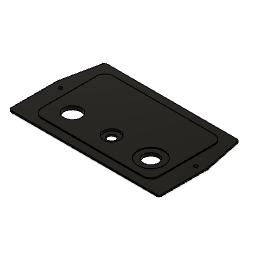
CableCover_Fusion (Autodesk Fusion 360 design; units mm, degrees)
Autodesk Fusion 360 part; units mm, degrees
sketch "Sketch1" plane through (0, 0, 0) normal (0, 1, 0) x (1, 0, 0)
  line L0 (-102.5, 67.5) -> (102.5, 67.5)
  line L1 (102.5, 67.5) -> (102.5, -67.5)
  line L2 (102.5, -67.5) -> (-102.5, -67.5)
  line L3 (-102.5, -67.5) -> (-102.5, 67.5)
  dimension "d1" = 205
  dimension "d2" = 135
  dimension "d3" = 67.5
  dimension "d4" = 102.5
  constraint horizontal L0
  constraint vertical L1
  constraint horizontal L2
  constraint vertical L3
  measures "d1" distance of L0.start L0.end
  measures "d2" distance of L0.start L2.end
  measures "d3" distance of origin L0
  measures "d4" distance of origin L1
  measures "d7" distance of L0.start
extrude "Extrude1" add sketch "Sketch1" along normal blind 10 makes body 1
sketch "Sketch2" plane through (0, 10, 0) normal (0, 1, 0) x (-1, 0, 0)
  line L0 (102.5, 67.5) -> (-102.5, 67.5)
  line L1 (-102.5, 67.5) -> (-102.5, -67.5)
  line L2 (-102.5, -67.5) -> (102.5, -67.5)
  line L3 (102.5, -67.5) -> (102.5, 67.5)
  line L4 (90, -55) -> (-90, -55)
  line L5 (-90, -55) -> (-90, 55)
  line L6 (-90, 55) -> (90, 55)
  line L7 (90, 55) -> (90, -55)
  dimension "d7" = 12.5
  dimension "d8" = 12.5
  dimension "d9" = 12.5
  dimension "d10" = 12.5
  constraint horizontal L4
  constraint vertical L5
  constraint horizontal L6
  constraint vertical L7
  measures "d7" distance of L3 L7
  measures "d8" distance of L1 L5
  measures "d9" distance of L2 L4
  measures "d10" distance of L0 L6
extrude "Extrude2" cut sketch "Sketch2" against normal blind 6 bodies 1
sketch "Sketch3" plane through (102.5, 0, 0) normal (1, 0, 0) x (0, 0, -1)
  line L0 (67.5, 4) -> (-67.5, 4)
  line L1 (-67.5, 4) -> (-67.5, 0)
  line L2 (-67.5, 0) -> (67.5, 0)
  line L3 (67.5, 0) -> (67.5, 4)
extrude "Extrude3" add sketch "Sketch3" along normal blind 12.5 bodies 1
extrude "Extrude4" add 1 faces at (-102.5, 1.3333, 22.5) along direction (-1, 0, 0) blind 12.5 on bodies 1 bodies 1
sketch "Sketch4" plane through (0, 4, 0) normal (0, 1, 0) x (-1, 0, 0)
  line L0 (-90, 55) -> (90, 55)
  line L1 (90, 55) -> (90, -55)
  line L2 (90, -55) -> (-90, -55)
  line L3 (-90, -55) -> (-90, 55)
  line L4 (115, 67.5) -> (-115, 67.5)
  line L5 (-115, 67.5) -> (-115, -67.5)
  line L6 (-115, -67.5) -> (115, -67.5)
  line L7 (115, -67.5) -> (115, 67.5)
  point P0 (103.5, 0)
  point P1 (-103.5, 0)
  dimension "d17" = 207
  dimension "d18" = 11.5
  dimension "d19" = 67.5
  dimension "d20" = 67.5
  measures "d17" horizontal distance of P0 P1
  measures "d18" distance of L7 P0
  measures "d19" distance of L4 P0
  measures "d20" distance of L4 P1
hole "Hole1" at (-103.5, 4, 0) at (103.5, 4, 0) direction (0, -1, 0) diameter 5.3 depth 4 tip angle 180 bodies 1
fillet "Fillet1" radius 12.5 4 edges at (-90, 7, -55) (-90, 7, 55) (90, 7, 55) (90, 7, -55) on bodies 1
sketch "Sketch5" plane through (0, 4, 0) normal (0, 1, 0) x (-1, 0, 0)
  circle A0 centre (103.5, 0) radius 2.65
  circle A1 centre (-103.5, 0) radius 2.65
  line L0 (90, 42.5) -> (90, -42.5)
  arc A2 (77.5, -55) -> (90, -42.5) centre (77.5, -42.5) ccw
  line L1 (77.5, -55) -> (-77.5, -55)
  arc A3 (-90, -42.5) -> (-77.5, -55) centre (-77.5, -42.5) ccw
  line L2 (-90, -42.5) -> (-90, 42.5)
  arc A4 (-77.5, 55) -> (-90, 42.5) centre (-77.5, 42.5) ccw
  line L3 (-77.5, 55) -> (77.5, 55)
  arc A5 (90, 42.5) -> (77.5, 55) centre (77.5, 42.5) ccw
  line L4 (115, 67.5) -> (-115, 67.5)
  line L5 (-115, 67.5) -> (-115, -67.5)
  line L6 (-115, -67.5) -> (115, -67.5)
  line L7 (115, -67.5) -> (115, 67.5)
  line L8 (102.5, -67.5) -> (-102.5, -67.5) construction
  line L9 (-102.5, -67.5) -> (-102.5, 67.5) construction
  line L10 (-102.5, 67.5) -> (102.5, 67.5) construction
  line L11 (102.5, 67.5) -> (102.5, -67.5) construction
  line L12 (-102.5, -67.5) -> (-115, -7.5)
  line L13 (102.5, -67.5) -> (115, -7.5)
  dimension "d28" = 135
  dimension "d29" = 205
  dimension "d30" = 12.5
  dimension "d32" = 60
  dimension "d33" = 60
  constraint horizontal L8
  constraint vertical L9
  constraint horizontal L10
  constraint vertical L11
  constraint collinear L6 L8
  constraint coincident L5 L12.end
  constraint coincident L7 L13.end
  measures "d28" distance of L8 L10
  measures "d29" distance of L9 L11
  measures "d30" distance of L7 L11
  measures "d32" distance of L5.end L12.end
  measures "d33" distance of L6.end L13.end
extrude "Extrude5" cut sketch "Sketch5" against normal up to surface (4 mm away) contours L6 L7 L13 | L5 L6 L12 bodies 1
fillet "Fillet3" radius 2 6 edges at (0, 0, -67.5) (108.75, 0, -37.5) (115, 0, 30) (0, 0, 67.5) (-115, 0, 30) (-108.75, 0, -37.5) on bodies 1
fillet "Fillet4" radius 4 12 edges at (102.0237, 0.5858, -66.9142) (102.5, 3, -67.5) (114.4142, 0.5858, -7.4396) (115, 3, -7.5) (114.4142, 0.5858, 66.9142) (115, 3, 67.5) (-102.0237, 0.5858, -66.9142) (-102.5, 3, -67.5) (-115, 3, -7.5) (-114.4142, 0.5858, -7.4396) (-115, 3, 67.5) (-114.4142, 0.5858, 66.9142) on bodies 1
extrude "Extrude6" cut 1 faces at (25.8333, 10, 18.3333) along direction (0, -1, 0) blind 4.5 on bodies 1 bodies 1
copy_body "CopyPasteBodies1" bodies 1 makes body 2
move_body "Move1" bodies 2 to x (1, 0, 0) y (0, 1, 0) z (0, 0, 1) at (0, 0, -150)
sketch "Sketch6" plane through (0, 5.5, 0) normal (0, 1, 0) x (-1, 0, 0)
  arc A0 (-90, -192.5) -> (-77.5, -205) centre (-77.5, -192.5) ccw
  line L0 (-77.5, -205) -> (77.5, -205)
  arc A1 (77.5, -205) -> (90, -192.5) centre (77.5, -192.5) ccw
  line L1 (90, -192.5) -> (90, -107.5)
  arc A2 (90, -107.5) -> (77.5, -95) centre (77.5, -107.5) ccw
  line L2 (77.5, -95) -> (-77.5, -95)
  arc A3 (-77.5, -95) -> (-90, -107.5) centre (-77.5, -107.5) ccw
  line L3 (-90, -107.5) -> (-90, -192.5)
  line L4 (60, -125) -> (-60, -125) construction
  point P0 (0, -125)
  dimension "d40" = 30
  dimension "d41" = 30
  dimension "d42" = 30
  constraint horizontal L4
  constraint midpoint L4 P0
  measures "d40" distance of L2 L4
  measures "d41" distance of L3 L4.end
  measures "d42" distance of L1 L4.start
hole "Hole2" at (60, 5.5, -125) direction (0, -1, 0) diameter 23 depth 5.5 tip angle 180 bodies 2
hole "Hole3" at (0, 5.5, -125) direction (0, -1, 0) diameter 13 depth 5.5 tip angle 180 bodies 2
hole "Hole4" at (-60, 5.5, -125) direction (0, -1, 0) diameter 26.5 depth 5.5 tip angle 180 bodies 2
hole "Hole5" at (60, 5.5, -125) direction (0, -1, 0) diameter 40 depth 1 tip angle 180 bodies 2
hole "Hole6" at (0, 5.5, -125) direction (0, -1, 0) diameter 25 depth 3 tip angle 180 bodies 2
move_body "Move2" bodies 2 to x (1, 0, 0) y (0, -1, 0) z (0, 0, -1) at (0, 0, -300)
move_body "Move3" bodies 2 to x (1, 0, 0) y (0, -1, 0) z (0, 0, -1) at (0, 0, -300)
hidden bodies 1
equation "d3 = ( 135 / 2 ) * 1 mm"
equation "d4 = ( 205 / 2 ) * 1 mm"
equation "d18 = ( ( 230 - 207 ) / 2 ) * 1 mm"
equation "d19 = ( 135 / 2 ) * 1 mm"
equation "d20 = ( 135 / 2 ) * 1 mm"
equation "d30 = ( 25 / 2 ) * 1 mm"
